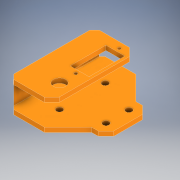
# Autodesk Inventor part: base 2.0 upload
Saved by Autodesk Inventor 2021 (Build 250183000, 183)
## iProperties
Created: 2021-03-12
Part Number: base 2.0 upload
Material: Generic
Document SubType Name: Modeling
Designer: Luthfi
Density: 1 g/cm^3
Appearance: Orange
Author: Luthfi
Autodesk Inventor part; units mm, degrees
ref_plane "YZ Plane" through (0, 0, 0) normal (1, 0, 0) x (0, 1, 0)
ref_plane "XZ Plane" through (0, 0, 0) normal (0, 1, 0) x (-1, 0, 0)
ref_plane "XY Plane" through (0, 0, 0) normal (0, 0, 1) x (1, 0, 0)
sketch "Sketch1" plane through (0, 0, 0) normal (0, 1, 0) x (-1, 0, 0)
  line L0 (0, 0) -> (37, 0)
  line L1 (57, -25.5) -> (57, -44.5)
  line L2 (37, -70) -> (0, -70)
  line L3 (0, -60) -> (0, -10)
  circle A0 centre (27, -20) radius 15 construction
  circle A1 centre (27, -50) radius 15 construction
  circle A2 centre (27, -20) radius 2
  circle A3 centre (27, -50) radius 2
  circle A4 centre (50, -27.5) radius 2
  circle A5 centre (50, -42.5) radius 2
  line L4 (50, -27.5) -> (50, -42.5) construction
  line L5 (27, -20) -> (50, -27.5) construction
  line L6 (25, 0) -> (0, -10)
  line L7 (0, -60) -> (25, -70)
  line L8 (37, 0) -> (57, -15)
  line L9 (57, -55) -> (37, -70)
  line L10 (7, -10) -> (7, -60)
  line L11 (43.6667, -5) -> (12, -5)
  line L12 (43.6667, -65) -> (12, -65)
  line L13 (12, -5) -> (7, -10)
  line L14 (7, -60) -> (12, -65)
  line L15 (32, -5) -> (47.5, -20.5)
  line L16 (47.5, -20.5) -> (52, -20.5)
  line L17 (57, -35) -> (0, -35) construction
  line L18 (32, -65) -> (47.5, -49.5)
  line L19 (47.5, -49.5) -> (52, -49.5)
  line L20 (52, -20.5) -> (57, -25.5)
  line L21 (57, -44.5) -> (52, -49.5)
  point P0 (57, -70)
  point P1 (57, 0)
  point P2 (48, 0)
  point P3 (57, -10)
  point P4 (57, -60)
  point P5 (38, -70)
  point P6 (57, -15)
  point P7 (57, -15)
  point P8 (7, -7.2)
  point P9 (7, -62.8)
  point P10 (7, -5)
  point P11 (7, -65)
  point P12 (7, -5)
  point P13 (7, -65)
  point P14 (57, -20.5)
  point P15 (57, -49.5)
  point P16 (32, -65)
  point P17 (57, -49.5)
  point P18 (57, -20.5)
  point P19 (57, -49.5)
  dimension "d47" = 0
  dimension "d0" = 57
  dimension "d7" = 30
  dimension "d8" = 30
  dimension "d12" = 4
  dimension "d13" = 4
  dimension "d17" = 4
  dimension "d18" = 4
  dimension "d19" = 15
  dimension "d21" = 7
  dimension "d36" = 27.5
  dimension "d38" = 25
  dimension "d40" = 25
  dimension "d52" = 30
  dimension "d90" = 15
  dimension "d91" = 20
  dimension "d92" = 15
  dimension "d93" = 20
  dimension "d124" = 70
  dimension "d132" = 7
  dimension "d133" = 5
  dimension "d134" = 5
  dimension "d135" = 5
  dimension "d136" = 5
  dimension "d137" = 5
  dimension "d138" = 5
  dimension "d139" = 45
  dimension "d140" = 15.5
  dimension "d141" = 7
  dimension "d142" = 5
  dimension "d143" = 5
  dimension "d144" = 5
  dimension "d145" = 5
  dimension "d146" = 25
  dimension "d165" = 15
  constraints: 42 end point, 31 point on line, 7 horizontal, 7 vertical, 6 centre point, 3 symmetric about line, 2 coincident, 2 perpendicular, 1 equal radius, 1 midpoint, 1 parallel, 47 other
  measures "d0" distance of point (57, -70) point (0, -70)
  measures "d7" diameter of A0
  measures "d8" diameter of A1
  measures "d12" diameter of A2
  measures "d13" diameter of A3
  measures "d17" diameter of A4
  measures "d18" diameter of A5
  measures "d19" distance of L4.start L4.end
  measures "d36" distance from line of L0 L4.start
  measures "d38" distance of point (0, 0) L6.start
  measures "d40" distance of point (0, -70) L7.end
  measures "d90" vertical distance of L8.start L8.end
  measures "d91" horizontal distance of L8.start L8.end
  measures "d92" vertical distance of L9.start L9.end
  measures "d93" horizontal distance of L9.start L9.end
  measures "d124" distance between parallel lines of L2 L0
  measures "d132" distance between parallel lines of L3 L10
  measures "d133" distance between parallel lines of L2 L12
  measures "d134" distance between parallel lines of L11 L0
  measures "d135" distance of L11.end point (7, -5)
  measures "d136" distance of L10.start point (7, -5)
  measures "d137" distance of L10.end point (7, -65)
  measures "d138" distance of L12.end point (7, -65)
  measures "d139" angle of L11 L15
  measures "d140" distance between parallel lines of L11 L16
  measures "d141" distance from line of L16 L4.start
  measures "d142" distance of L16.end point (57, -20.5)
  measures "d143" distance of L20.end point (57, -20.5)
  measures "d144" distance of L21.start point (57, -49.5)
  measures "d145" distance of L19.end point (57, -49.5)
  measures "d165" distance from line of L17 A0.centre
extrude "Extrusion1" add sketch "Sketch1" along normal blind 3 contours L11 L15 L16 L20 L1 L21 L19 L18 L12 L7 L14 L10 L13 L6 | L6 L13 L11 | L7 L12 L14
sketch "Sketch4" plane through (0, 3, 0) normal (0, 1, 0) x (1, 0, 0)
  line L0 (-33.2, 8.95) -> (-33.2, 41.25)
  line L1 (-33.2, 41.25) -> (-20.8, 41.25)
  line L2 (-20.8, 41.25) -> (-20.8, 8.95)
  line L3 (-20.8, 8.95) -> (-33.2, 8.95)
  line L4 (-33.2, 13.35) -> (-20.8, 13.35)
  line L5 (-33.2, 36.85) -> (-20.8, 36.85)
  circle A0 centre (-27, 20) radius 2.45
  circle A1 centre (-27, 20) radius 2 projected
  circle A2 centre (-27, 20) radius 16.1 construction
  circle A3 centre (-27, 50) radius 2 projected
  circle A4 centre (-27, 50) radius 16.1 construction
  line L6 (-27, 8.95) -> (-27, 13.35) construction
  line L7 (-27, 41.25) -> (-27, 36.85) construction
  circle A5 centre (-27, 10.85) radius 1
  circle A6 centre (-27, 39.35) radius 1
  circle A7 centre (-27, 20) radius 2 projected
  circle A8 centre (-27, 20) radius 9.85 construction
  line L8 (-57, 44.5) -> (-57, 25.5) projected
  line L9 (-32, 5) -> (-12, 5) projected
  line L10 (-12, 65) -> (-32, 65) projected
  line L11 (-12, 5) -> (-10, 7) projected
  line L12 (-10, 63) -> (-12, 65) projected
  line L13 (-32, 65) -> (-47.5, 49.5) projected
  line L14 (-47.5, 49.5) -> (-52, 49.5) projected
  line L15 (-52, 20.5) -> (-47.5, 20.5) projected
  line L16 (-47.5, 20.5) -> (-32, 5) projected
  line L17 (-52, 49.5) -> (-57, 44.5) projected
  line L18 (-57, 25.5) -> (-52, 20.5) projected
  line L19 (-10, 7) -> (-10, 63) projected
  point P0 (0, 0)
  point P1 (-22.9289, 0)
  point P2 (-27.9289, 0)
  dimension "d22" = 32.3
  dimension "d23" = 12.4
  dimension "d24" = 4.4
  dimension "d25" = 4.4
  dimension "d27" = 6.2
  dimension "d28" = 11.05
  dimension "d49" = 32.2
  dimension "d50" = 32.2
  dimension "d53" = 4.9
  dimension "d54" = 2.2
  dimension "d57" = 2
  dimension "d58" = 2
  dimension "d59" = 1.9
  dimension "d60" = 1.9
  dimension "d87" = 19.7
  constraints: 16 end point, 6 centre point, 6 point on line, 4 coincident, 4 midpoint, 2 parallel, 2 perpendicular
  measures "d22" distance between parallel lines of L1 L3
  measures "d23" distance between parallel lines of L2 L0
  measures "d24" distance between parallel lines of L1 L5
  measures "d25" distance between parallel lines of L3 L4
  measures "d27" distance from line of L0 A0.centre
  measures "d28" distance from line of L3 A0.centre
  measures "d49" diameter of A2
  measures "d50" diameter of A4
  measures "d53" diameter of A0
  measures "d57" diameter of A5
  measures "d58" diameter of A6
  measures "d59" distance from line of L1 A6.centre
  measures "d60" distance from line of L3 A5.centre
  measures "d87" diameter of A8
sketch "Sketch10" plane through (0, 3, 0) normal (0, 1, 0) x (1, 0, 0)
  line L0 (-12, 5) -> (-7, 10) projected
  line L1 (-10, 7) -> (-10, 63)
  line L2 (-7, 60) -> (-12, 65) projected
  line L3 (-7, 10) -> (-7, 60) projected
  line L4 (-7, 60) -> (-12, 65) projected
  line L5 (-47.5, 20.5) -> (-32, 5) projected
  line L6 (-32, 65) -> (-47.5, 49.5) projected
  line L7 (-32, 5) -> (-12, 5) projected
  line L8 (-12, 65) -> (-32, 65) projected
  line L9 (-12, 65) -> (-32, 65) projected
  point P0 (0, 0)
  dimension "d147" = 3
  constraints: 3 point on line, 2 end point, 1 vertical
  measures "d147" distance between parallel lines of L3 L1
extrude "Extrusion7" add sketch "Sketch10" along normal blind 15.1
sketch "Sketch11" plane through (0, 18.1, 0) normal (0, 1, 0) x (1, 0, 0)
  line L0 (-12, 5) -> (-10, 7) projected
  line L1 (-10, 7) -> (-30, 7)
  line L2 (-35, 12) -> (-35, 58.0775)
  line L3 (-30, 63.0775) -> (-10, 63.0775)
  line L4 (-10, 63.0775) -> (-10, 7)
  line L5 (-30, 7) -> (-35, 12)
  line L6 (-35, 58.0775) -> (-30, 63.0775)
  circle A0 centre (-27, 10.85) radius 1 projected
  circle A1 centre (-27, 39.35) radius 1 projected
  line L7 (-20.8, 8.95) -> (-33.2, 8.95) projected
  line L8 (-33.2, 8.95) -> (-33.2, 41.25) projected
  line L9 (-33.2, 36.85) -> (-20.8, 36.85) projected
  line L10 (-33.2, 41.25) -> (-20.8, 41.25) projected
  line L11 (-20.8, 41.25) -> (-20.8, 8.95) projected
  line L12 (-33.2, 13.35) -> (-20.8, 13.35) projected
  circle A2 centre (-27, 50) radius 2 projected
  circle A3 centre (-27, 50) radius 4
  point P0 (0, 0)
  point P1 (-35, 63.0775)
  point P2 (-35, 7)
  dimension "d150" = 25
  dimension "d151" = 56.0775
  dimension "d152" = 5
  dimension "d153" = 5
  dimension "d154" = 5
  dimension "d155" = 5
  dimension "d156" = 8
  constraints: 12 end point, 4 point on line, 2 parallel, 1 centre point, 1 coincident, 1 horizontal, 1 perpendicular
  measures "d150" distance between parallel lines of L4 L2
  measures "d151" distance between parallel lines of L1 L3
  measures "d152" distance of L1.end point (-35, 7)
  measures "d153" distance of L2.start point (-35, 7)
  measures "d154" distance of L2.end point (-35, 63.077)
  measures "d155" distance of L3.start point (-35, 63.077)
  measures "d156" diameter of A3
extrude "Extrusion8" add sketch "Sketch11" against normal blind 3 contours L1 L5 L7 L11 L10 L8 L2 L6 L3 L4 | L5 L8 L12 L11 L7 | L8 L10 L11 L9
body "Solid1"
